Autodesk Inventor part; units mm, degrees
(part 2 of 3)
  line L789 (-22.603724, 22.825849) -> (-22.585944, 20.520291)
  line L790 (-22.585944, 20.520291) -> (-22.128744, 18.275693)
  line L791 (-22.128744, 18.275693) -> (-21.252444, 16.160381)
  line L792 (-21.252444, 16.160381) -> (-19.979904, 14.236585)
  line L793 (-19.979904, 14.236585) -> (-18.328904, 12.570599)
  line L794 (-18.328904, 12.570599) -> (-16.850624, 11.507863)
  line L795 (-16.850624, 11.507863) -> (-16.317224, 11.225415)
  line L796 (7.322556, -11.331563) -> (7.640056, -11.842865)
  line L797 (7.640056, -11.842865) -> (8.788136, -13.249517)
  line L798 (8.788136, -13.249517) -> (10.561056, -14.792059)
  line L799 (10.561056, -14.792059) -> (12.560036, -15.938615)
  line L800 (12.560036, -15.938615) -> (14.726656, -16.675469)
  line L801 (14.726656, -16.675469) -> (16.994876, -16.988397)
  line L802 (16.994876, -16.988397) -> (19.298656, -16.860381)
  line L803 (19.298656, -16.860381) -> (21.569416, -16.274657)
  line L804 (21.569416, -16.274657) -> (23.233116, -15.534501)
  line L805 (23.233116, -15.534501) -> (23.746196, -15.218779)
  line L806 (23.746196, -15.218779) -> (24.254196, -14.903311)
  line L807 (24.254196, -14.903311) -> (25.663896, -13.748373)
  line L808 (25.663896, -13.748373) -> (27.203136, -11.980787)
  line L809 (27.203136, -11.980787) -> (28.351216, -9.979775)
  line L810 (28.351216, -9.979775) -> (29.087816, -7.811885)
  line L811 (29.087816, -7.811885) -> (29.402776, -5.543919)
  line L812 (29.402776, -5.543919) -> (29.275776, -3.240901)
  line L813 (29.275776, -3.240901) -> (28.689036, -0.968617)
  line L814 (28.689036, -0.968617) -> (27.947356, 0.693305)
  line L815 (27.947356, 0.693305) -> (27.629856, 1.204353)
  line L816 (27.629856, 1.204353) -> (27.317436, 1.716925)
  line L817 (27.317436, 1.716925) -> (26.164276, 3.124339)
  line L818 (26.164276, 3.124339) -> (24.396436, 4.666119)
  line L819 (24.396436, 4.666119) -> (22.392376, 5.812675)
  line L820 (22.392376, 5.812675) -> (20.225756, 6.550037)
  line L821 (20.225756, 6.550037) -> (17.957536, 6.862711)
  line L822 (17.957536, 6.862711) -> (15.653756, 6.734441)
  line L823 (15.653756, 6.734441) -> (13.382996, 6.148971)
  line L824 (13.382996, 6.148971) -> (11.721836, 5.407291)
  line L825 (11.721836, 5.407291) -> (11.208756, 5.092077)
  line L826 (11.208756, 5.092077) -> (10.698216, 4.776355)
  line L827 (10.698216, 4.776355) -> (9.291056, 3.622941)
  line L828 (9.291056, 3.622941) -> (7.749276, 1.854847)
  line L829 (7.749276, 1.854847) -> (6.601196, -0.145911)
  line L830 (6.601196, -0.145911) -> (5.864596, -2.313547)
  line L831 (5.864596, -2.313547) -> (5.549636, -4.581767)
  line L832 (5.549636, -4.581767) -> (5.676636, -6.885801)
  line L833 (5.676636, -6.885801) -> (6.263376, -9.157069)
  line L834 (6.263376, -9.157069) -> (7.007596, -10.818991)
  line L835 (7.007596, -10.818991) -> (7.322556, -11.331563)
  line L836 (9.164056, -42.734345) -> (9.174216, -43.335055)
  line L837 (9.174216, -43.335055) -> (9.458696, -45.132105)
  line L838 (9.458696, -45.132105) -> (10.210536, -47.354859)
  line L839 (10.210536, -47.354859) -> (11.358616, -49.355871)
  line L840 (11.358616, -49.355871) -> (12.857216, -51.085103)
  line L841 (12.857216, -51.085103) -> (14.660616, -52.500442)
  line L842 (14.660616, -52.500442) -> (16.712936, -53.550503)
  line L843 (16.712936, -53.550503) -> (18.965916, -54.192641)
  line L844 (18.965916, -54.192641) -> (20.776936, -54.391091)
  line L845 (20.776936, -54.391091) -> (21.378916, -54.377324)
  line L846 (21.378916, -54.377324) -> (21.978356, -54.36216)
  line L847 (21.978356, -54.36216) -> (23.779216, -54.076893)
  line L848 (23.779216, -54.076893) -> (26.001716, -53.327263)
  line L849 (26.001716, -53.327263) -> (27.998156, -52.179361)
  line L850 (27.998156, -52.179361) -> (29.730436, -50.679973)
  line L851 (29.730436, -50.679973) -> (31.145216, -48.878859)
  line L852 (31.145216, -48.878859) -> (32.196776, -46.825777)
  line L853 (32.196776, -46.825777) -> (32.836856, -44.569749)
  line L854 (32.836856, -44.569749) -> (33.034976, -42.760507)
  line L855 (33.034976, -42.760507) -> (33.022276, -42.159543)
  line L856 (33.022276, -42.159543) -> (33.007036, -41.557309)
  line L857 (33.007036, -41.557309) -> (32.722556, -39.760513)
  line L858 (32.722556, -39.760513) -> (31.973256, -37.537759)
  line L859 (31.973256, -37.537759) -> (30.822636, -35.538017)
  line L860 (30.822636, -35.538017) -> (29.324036, -33.807261)
  line L861 (29.324036, -33.807261) -> (27.520636, -32.393497)
  line L862 (27.520636, -32.393497) -> (25.470856, -31.342191)
  line L863 (25.470856, -31.342191) -> (23.215336, -30.699825)
  line L864 (23.215336, -30.699825) -> (21.404316, -30.501451)
  line L865 (21.404316, -30.501451) -> (20.804876, -30.516691)
  line L866 (20.804876, -30.516691) -> (20.202896, -30.530407)
  line L867 (20.202896, -30.530407) -> (18.407116, -30.815395)
  line L868 (18.407116, -30.815395) -> (16.184616, -31.565203)
  line L869 (16.184616, -31.565203) -> (14.183096, -32.713029)
  line L870 (14.183096, -32.713029) -> (12.450816, -34.212391)
  line L871 (12.450816, -34.212391) -> (11.036036, -36.013759)
  line L872 (11.036036, -36.013759) -> (9.984476, -38.066841)
  line L873 (9.984476, -38.066841) -> (9.346936, -40.322869)
  line L874 (9.346936, -40.322869) -> (9.146276, -42.132111)
  line L875 (9.146276, -42.132111) -> (9.164056, -42.734345)
  line L876 (-33.408884, -56.423701) -> (-34.033724, -57.046585)
  line L877 (-34.033724, -57.046585) -> (-36.157164, -58.665759)
  line L878 (-36.157164, -58.665759) -> (-39.200084, -60.267051)
  line L879 (-39.200084, -60.267051) -> (-42.443664, -61.227526)
  line L880 (-42.443664, -61.227526) -> (-45.786304, -61.548633)
  line L881 (-45.786304, -61.548633) -> (-49.128944, -61.227526)
  line L882 (-49.128944, -61.227526) -> (-52.369984, -60.267051)
  line L883 (-52.369984, -60.267051) -> (-55.415444, -58.665759)
  line L884 (-55.415444, -58.665759) -> (-57.536344, -57.046585)
  line L885 (-57.536344, -57.046585) -> (-58.158644, -56.423701)
  line L886 (-58.158644, -56.423701) -> (-58.783484, -55.799445)
  line L887 (-58.783484, -55.799445) -> (-60.404004, -53.677275)
  line L888 (-60.404004, -53.677275) -> (-62.004204, -50.634507)
  line L889 (-62.004204, -50.634507) -> (-62.964324, -47.390673)
  line L890 (-62.964324, -47.390673) -> (-63.286904, -44.048795)
  line L891 (-63.286904, -44.048795) -> (-62.964324, -40.705901)
  line L892 (-62.964324, -40.705901) -> (-62.004204, -37.463337)
  line L893 (-62.004204, -37.463337) -> (-60.404004, -34.419147)
  line L894 (-60.404004, -34.419147) -> (-58.783484, -32.297231)
  line L895 (-58.783484, -32.297231) -> (-58.158644, -31.674169)
  line L896 (-58.158644, -31.674169) -> (-57.536344, -31.049837)
  line L897 (-57.536344, -31.049837) -> (-55.415444, -29.430841)
  line L898 (-55.415444, -29.430841) -> (-52.369984, -27.829625)
  line L899 (-52.369984, -27.829625) -> (-49.128944, -26.868997)
  line L900 (-49.128944, -26.868997) -> (-45.786304, -26.547941)
  line L901 (-45.786304, -26.547941) -> (-42.443664, -26.868997)
  line L902 (-42.443664, -26.868997) -> (-39.200084, -27.829625)
  line L903 (-39.200084, -27.829625) -> (-36.157164, -29.430841)
  line L904 (-36.157164, -29.430841) -> (-34.033724, -31.049837)
  line L905 (-34.033724, -31.049837) -> (-33.408884, -31.674169)
  line L906 (-33.408884, -31.674169) -> (-32.789124, -32.297231)
  line L907 (-32.789124, -32.297231) -> (-31.168604, -34.419147)
  line L908 (-31.168604, -34.419147) -> (-29.568404, -37.463337)
  line L909 (-29.568404, -37.463337) -> (-28.605744, -40.705901)
  line L910 (-28.605744, -40.705901) -> (-28.283164, -44.048795)
  line L911 (-28.283164, -44.048795) -> (-28.605744, -47.390673)
  line L912 (-28.605744, -47.390673) -> (-29.568404, -50.634507)
  line L913 (-29.568404, -50.634507) -> (-31.168604, -53.677275)
  line L914 (-31.168604, -53.677275) -> (-32.789124, -55.799445)
  line L915 (-32.789124, -55.799445) -> (-33.408884, -56.423701)
  line L916 (-54.188624, -52.523861) -> (-53.591724, -51.928561)
  line L917 (-52.384423, -50.722098) -> (-38.507387, -36.843538)
  line L918 (-37.907224, -36.242359) -> (-37.307784, -35.645713)
  line L919 (-37.307784, -52.523861) -> (-37.907224, -51.928561)
  line L920 (-39.111184, -50.721375) -> (-52.989744, -36.844339)
  line L921 (-53.591724, -36.242359) -> (-54.188624, -35.645713)
  line L922 (14.729196, -13.081623) -> (14.482816, -13.060795)
  line L923 (18.978616, -13.034887) -> (18.920196, -13.036157)
  line L924 (18.920196, -13.036157) -> (18.783036, -13.040475)
  line L925 (18.783036, -13.040475) -> (17.419056, -13.063589)
  line L926 (17.419056, -13.063589) -> (17.284436, -13.066637)
  line L927 (17.284436, -13.066637) -> (17.068536, -13.066637)
  line L928 (17.068536, -13.066637) -> (14.942556, -13.099657)
  line L929 (14.942556, -13.099657) -> (14.729196, -13.081623)
  line L930 (-4.793244, -62.273498) -> (-4.752604, -62.254194)
  line L931 (-4.752604, -62.254194) -> (-4.559564, -62.083303)
  line L932 (-4.559564, -62.083303) -> (-4.559564, -62.026814)
  line L933 (-4.559564, -62.026814) -> (-4.559564, -61.924833)
  line L934 (-4.559564, -61.924833) -> (-4.592584, -61.734663)
  line L935 (-52.737996, -50.368564) -> (-38.86096, -36.490004)
  line L936 (-52.03085, -51.075632) -> (-38.153814, -37.197072)
  line L937 (-39.464718, -51.074948) -> (-53.343278, -37.197912)
  line L938 (-38.75765, -50.367802) -> (-52.63621, -36.490766)
  line L939 (-38.153814, -37.197072) -> (-38.86096, -36.490004)
  line L940 (-38.75765, -50.367802) -> (-39.464718, -51.074948)
  line L941 (-52.737996, -50.368564) -> (-52.03085, -51.075632)
  line L942 (-52.63621, -36.490766) -> (-53.343278, -37.197912)
  point P0 (26.657089, 2.522869)
  point P1 (28.23602, 0.046481)
  point P2 (-70.980287, -13.221606)
  point P3 (-70.781416, -10.664974)
  point P4 (-12.499708, 33.522102)
  point P5 (3.750981, -66.644317)
  point P6 (-70.90252, -13.99275)
  point P7 (-14.451188, -45.049937)
  point P8 (-14.090958, -45.024663)
  point P9 (-13.657176, -45.024663)
  point P10 (-12.392664, -45.113647)
  point P11 (-11.715458, -45.204164)
  point P12 (-10.362386, -45.543008)
  point P13 (-9.292197, -45.87547)
  point P14 (-8.154694, -46.428219)
  point P15 (-7.207823, -46.941879)
  point P16 (-6.157427, -47.746057)
  point P17 (-5.380475, -48.386819)
  point P18 (-4.4666, -49.432156)
  point P19 (-3.865434, -50.160677)
  point P20 (-3.113204, -51.481774)
  point P21 (-2.717481, -52.211101)
  point P22 (-2.17304, -53.8869)
  point P23 (-1.982369, -54.500406)
  point P24 (-1.79223, -55.839475)
  point P25 (-1.848254, -58.490356)
  point P26 (-2.230518, -60.213444)
  point P27 (-2.494622, -61.063215)
  point P28 (-4.038829, -63.964888)
  point P29 (-4.410069, -64.414728)
  point P30 (-6.724497, -66.636927)
  point P31 (-6.901029, -66.782518)
  point P32 (-9.069068, -67.970607)
  point P33 (-10.477781, -68.408219)
  point P34 (-16.530305, -68.504563)
  point P35 (-18.074437, -68.024885)
  point P36 (-18.440429, -67.879534)
  point P37 (-19.879408, -67.099838)
  point P38 (-20.383214, -66.812521)
  point P39 (-22.021991, -65.457083)
  point P40 (-22.425656, -64.997007)
  point P41 (-23.403552, -63.814127)
  point P42 (-23.833695, -63.116856)
  point P43 (-24.482688, -61.917917)
  point P44 (-24.794771, -61.149472)
  point P45 (-25.204455, -59.836085)
  point P46 (-25.430368, -58.777249)
  point P47 (-25.521621, -58.095078)
  point P48 (-25.593304, -57.024666)
  point P49 (-25.593304, -56.661836)
  point P50 (-25.56963, -56.17919)
  point P51 (-25.419783, -55.059031)
  point P52 (-25.301336, -54.389917)
  point P53 (-24.905044, -53.119435)
  point P54 (-24.588154, -52.192295)
  point P55 (-24.111863, -51.312447)
  point P56 (-21.065728, -47.667296)
  point P57 (-20.493311, -47.193856)
  point P58 (-19.456689, -46.586467)
  point P59 (-18.526645, -46.082568)
  point P60 (-17.578172, -45.736339)
  point P61 (-16.261766, -45.327388)
  point P62 (-15.697902, -45.216811)
  point P63 (-32.132489, 34.644603)
  point P64 (-35.142865, 34.293968)
  point P65 (-69.1257, 0.22919)
  point P66 (-70.299173, -6.530143)
  point P67 (-70.363625, -7.082766)
  point P68 (15.877196, -62.416221)
  point P69 (17.047598, -61.83976)
  point P70 (34.387532, -28.646734)
  point P71 (34.353637, -28.003816)
  point P72 (9.452137, 19.037752)
  point P73 (8.27439, 20.009449)
  point P74 (-36.407377, 19.257413)
  point P75 (-37.127948, 15.741932)
  point P76 (-37.16308, 15.662676)
  point P77 (-38.109165, 13.74007)
  point P78 (-38.289337, 13.473296)
  point P79 (-39.40199, 12.011768)
  point P80 (-39.793143, 11.604587)
  point P81 (-40.934583, 10.582054)
  point P82 (-41.579317, 10.105711)
  point P83 (-42.720858, 9.425909)
  point P84 (-43.526766, 9.019144)
  point P85 (-44.809198, 8.564772)
  point P86 (-45.680707, 8.299855)
  point P87 (-46.652701, 8.12955)
  point P88 (-47.350022, 8.023598)
  point P89 (-47.938503, 7.999615)
  point P90 (-48.575756, 7.994027)
  point P91 (-49.709686, 8.101058)
  point P92 (-50.388844, 8.190593)
  point P93 (-51.657409, 8.529209)
  point P94 (-52.659665, 8.831052)
  point P95 (-53.784254, 9.384239)
  point P96 (-54.690294, 9.860171)
  point P97 (-55.678233, 10.610482)
  point P98 (-56.476925, 11.244335)
  point P99 (-57.323583, 12.191296)
  point P100 (-57.971801, 12.941087)
  point P101 (-58.65977, 14.095394)
  point P102 (-59.126949, 14.900308)
  point P103 (-59.690576, 16.492921)
  point P104 (-59.895339, 17.084166)
  point P105 (-60.235804, 19.618519)
  point P106 (-60.199445, 20.635684)
  point P107 (-60.139424, 21.274863)
  point P108 (-44.404458, 31.181517)
  point P109 (-43.908, 31.00537)
  point P110 (-42.823468, 30.47202)
  point P111 (-41.847578, 29.942526)
  point P112 (-40.939105, 29.251808)
  point P113 (-40.093943, 28.56811)
  point P114 (-39.285921, 27.663664)
  point P115 (-38.623993, 26.888971)
  point P116 (-37.922645, 25.712215)
  point P117 (-37.482851, 24.950917)
  point P118 (-36.898866, 23.305176)
  point P119 (-36.384985, 20.504957)
  point P120 (-36.383619, 20.472644)
  point P121 (0.598463, 25.558408)
  point P122 (1.111089, 23.222486)
  point P123 (1.165157, 21.742405)
  point P124 (1.172107, 20.840768)
  point P125 (0.899345, 19.25247)
  point P126 (0.747134, 18.449733)
  point P127 (0.310087, 17.242941)
  point P128 (0.104117, 16.687319)
  point P129 (-0.468312, 15.612618)
  point P130 (-0.902103, 15.008527)
  point P131 (-1.849187, 13.821679)
  point P132 (-2.505593, 13.172266)
  point P133 (-4.28973, 11.767595)
  point P134 (-4.848146, 11.398244)
  point P135 (-7.446953, 10.303356)
  point P136 (-8.75938, 10.036862)
  point P137 (-9.575058, 9.890829)
  point P138 (-12.609908, 10.030609)
  point P139 (-14.415298, 10.433739)
  point P140 (-14.788027, 10.572332)
  point P141 (-17.365174, 11.877773)
  point P142 (-19.365663, 13.616768)
  point P143 (-22.450919, 23.631804)
  point P144 (-21.72057, 26.328829)
  point P145 (-19.675191, 29.606141)
  point P146 (-18.975433, 30.299284)
  point P147 (-17.882197, 31.264757)
  point P148 (-16.576816, 32.129378)
  point P149 (-16.244236, 32.331452)
  point P150 (-15.367761, 32.6933)
  point P151 (29.198236, -7.016772)
  point P152 (28.443584, -9.707927)
  point P153 (27.76169, -11.007272)
  point P154 (27.305264, -11.802786)
  point P155 (26.260434, -13.063339)
  point P156 (25.715234, -13.689419)
  point P157 (24.776107, -14.47572)
  point P158 (21.082473, -16.40026)
  point P159 (19.905491, -16.703853)
  point P160 (18.941227, -16.880243)
  point P161 (15.34623, -16.760947)
  point P162 (14.597597, -16.631577)
  point P163 (14.035431, -16.440388)
  point P164 (11.968166, -15.599136)
  point P165 (11.229638, -15.175538)
  point P166 (9.490883, -13.860947)
  point P167 (8.941532, -13.382981)
  point P168 (7.614367, -11.801495)
  point P169 (7.165811, -11.076474)
  point P170 (6.963602, -10.720747)
  point P171 (6.517957, -9.725576)
  point P172 (6.225389, -9.010022)
  point P173 (5.995587, -8.120458)
  point P174 (5.664674, -6.668788)
  point P175 (5.656568, -6.521727)
  point P176 (8.809351, 3.070527)
  point P177 (9.246444, 3.57178)
  point P178 (9.815194, 4.052564)
  point P179 (10.647556, 4.73483)
  point P180 (11.165512, 5.065335)
  point P181 (11.589468, 5.325969)
  point P182 (13.830183, 6.264269)
  point P183 (14.964707, 6.556783)
  point P184 (16.016046, 6.754612)
  point P185 (19.962259, 6.58636)
  point P186 (20.621162, 6.415469)
  point P187 (28.298949, -51.919007)
  point P188 (27.202918, -52.636602)
  point P189 (25.423153, -53.522407)
  point P190 (24.575291, -53.808384)
  point P191 (22.13415, -54.337482)
  point P192 (21.979406, -54.361994)
  point P193 (20.689085, -54.381464)
  point P194 (19.560515, -54.257796)
  point P195 (18.877281, -54.167378)
  point P196 (17.574428, -53.796043)
  point P197 (16.628337, -53.507219)
  point P198 (15.440099, -52.899261)
  point P199 (14.594831, -52.448813)
  dimension "d36" = 0.5
  dimension "d37" = 0.5
  dimension "d38" = 0.5
  dimension "d39" = 0.5
  constraints: 1886 end point, 4 parallel, 4 perpendicular
  measures "d36" distance between parallel lines of L917 L935
  measures "d37" distance between parallel lines of L917 L936
  measures "d38" distance between parallel lines of L920 L937
  measures "d39" distance between parallel lines of L920 L938
sketch "Sketch1 outline for Extrusion3" plane through (0, 0, 0) normal (1, 0, 0) x (0, 1, 0)
  line L0 (-8.194304, 39.472755) -> (-13.782304, 40.987103)
  line L1 (-13.782304, 40.987103) -> (-19.456664, 41.986085)
  line L2 (-19.456664, 41.986085) -> (-25.166584, 42.447603)
  line L3 (-25.166584, 42.447603) -> (-30.851104, 42.347019)
  line L4 (-30.851104, 42.347019) -> (-36.469584, 41.662235)
  line L5 (-36.469584, 41.662235) -> (-41.958524, 40.369883)
  line L6 (-41.958524, 40.369883) -> (-47.272204, 38.443293)
  line L7 (-47.272204, 38.443293) -> (-52.354744, 35.861891)
  line L8 (-52.354744, 35.861891) -> (-57.155344, 32.600277)
  line L9 (-57.155344, 32.600277) -> (-60.571644, 29.694009)
  line L10 (-60.571644, 29.694009) -> (-61.618124, 28.635591)
  line L11 (-61.618124, 28.635591) -> (-62.369964, 27.748115)
  line L12 (-62.369964, 27.748115) -> (-64.437524, 24.924905)
  line L13 (-64.437524, 24.924905) -> (-66.926724, 20.862175)
  line L14 (-66.926724, 20.862175) -> (-69.085724, 16.492359)
  line L15 (-69.085724, 16.492359) -> (-70.922144, 11.855589)
  line L16 (-70.922144, 11.855589) -> (-72.438524, 6.993521)
  line L17 (-72.438524, 6.993521) -> (-73.637404, 1.946033)
  line L18 (-73.637404, 1.946033) -> (-74.521324, -3.242425)
  line L19 (-74.521324, -3.242425) -> (-75.095364, -8.532737)
  line L20 (-75.095364, -8.532737) -> (-75.362064, -13.882231)
  line L21 (-75.362064, -13.882231) -> (-75.329044, -19.251029)
  line L22 (-75.329044, -19.251029) -> (-74.993764, -24.596459)
  line L23 (-74.993764, -24.596459) -> (-74.363844, -29.878389)
  line L24 (-74.363844, -29.878389) -> (-73.441824, -35.053131)
  line L25 (-73.441824, -35.053131) -> (-72.230244, -40.081569)
  line L26 (-72.230244, -40.081569) -> (-70.731644, -44.921285)
  line L27 (-70.731644, -44.921285) -> (-69.441324, -48.395243)
  line L28 (-69.441324, -48.395243) -> (-68.953644, -49.530877)
  line L29 (-68.953644, -49.530877) -> (-68.570104, -50.426481)
  line L30 (-68.570104, -50.426481) -> (-67.221364, -53.028203)
  line L31 (-67.221364, -53.028203) -> (-65.128404, -56.283137)
  line L32 (-65.128404, -56.283137) -> (-62.702704, -59.270736)
  line L33 (-62.702704, -59.270736) -> (-59.969664, -61.964812)
  line L34 (-59.969664, -61.964812) -> (-56.959764, -64.341922)
  line L35 (-56.959764, -64.341922) -> (-53.695864, -66.375903)
  line L36 (-53.695864, -66.375903) -> (-50.208444, -68.044709)
  line L37 (-50.208444, -68.044709) -> (-47.455084, -69.056162)
  line L38 (-47.455084, -69.056162) -> (-46.517824, -69.322125)
  line L39 (-46.517824, -69.322125) -> (-45.420544, -69.633606)
  line L40 (-45.420544, -69.633606) -> (-42.082984, -70.421793)
  line L41 (-42.082984, -70.421793) -> (-37.378904, -71.292734)
  line L42 (-37.378904, -71.292734) -> (-32.453844, -71.932153)
  line L43 (-32.453844, -71.932153) -> (-27.361144, -72.340026)
  line L44 (-27.361144, -72.340026) -> (-22.146524, -72.515058)
  line L45 (-22.146524, -72.515058) -> (-16.860784, -72.457197)
  line L46 (-16.860784, -72.457197) -> (-11.554724, -72.16502)
  line L47 (-11.554724, -72.16502) -> (-6.284224, -71.638631)
  line L48 (-6.284224, -71.638631) -> (-1.092464, -70.875183)
  line L49 (-1.092464, -70.875183) -> (3.969756, -69.877496)
  line L50 (3.969756, -69.877496) -> (8.849096, -68.641405)
  line L51 (8.849096, -68.641405) -> (13.494756, -67.168282)
  line L52 (13.494756, -67.168282) -> (17.863556, -65.455356)
  line L53 (17.863556, -65.455356) -> (21.894536, -63.504078)
  line L54 (21.894536, -63.504078) -> (25.547056, -61.312972)
  line L55 (25.547056, -61.312972) -> (28.000696, -59.535328)
  line L56 (28.000696, -59.535328) -> (28.767776, -58.882116)
  line L57 (28.767776, -58.882116) -> (29.755836, -57.854102)
  line L58 (29.755836, -57.854102) -> (32.450776, -54.506864)
  line L59 (32.450776, -54.506864) -> (35.420036, -49.840757)
  line L60 (35.420036, -49.840757) -> (37.706036, -44.926619)
  line L61 (37.706036, -44.926619) -> (39.346876, -39.811313)
  line L62 (39.346876, -39.811313) -> (40.370496, -34.537511)
  line L63 (40.370496, -34.537511) -> (40.814996, -29.152457)
  line L64 (40.814996, -29.152457) -> (40.713396, -23.700601)
  line L65 (40.713396, -23.700601) -> (40.091096, -18.228679)
  line L66 (40.091096, -18.228679) -> (38.991276, -12.778347)
  line L67 (38.991276, -12.778347) -> (37.441876, -7.398373)
  line L68 (37.441876, -7.398373) -> (35.475916, -2.131937)
  line L69 (35.475916, -2.131937) -> (33.131496, 2.976765)
  line L70 (33.131496, 2.976765) -> (30.439096, 7.879727)
  line L71 (30.439096, 7.879727) -> (27.429196, 12.533515)
  line L72 (27.429196, 12.533515) -> (24.139896, 16.892155)
  line L73 (24.139896, 16.892155) -> (21.521156, 19.942949)
  line L74 (21.521156, 19.942949) -> (20.599136, 20.910435)
  line L75 (20.599136, 20.910435) -> (19.661876, 21.984093)
  line L76 (19.661876, 21.984093) -> (16.629116, 25.015583)
  line L77 (16.629116, 25.015583) -> (12.257776, 28.747097)
  line L78 (12.257776, 28.747097) -> (7.535916, 32.082371)
  line L79 (7.535916, 32.082371) -> (2.519416, 34.996513)
  line L80 (2.519416, 34.996513) -> (-2.738384, 37.468949)
  line L81 (-2.738384, 37.468949) -> (-8.194304, 39.472755)
extrude "Extrusion3" add sketch "Sketch1 outline for Extrusion3" along normal blind 0.25
sketch "Sketch1 outline for Extrusion17" plane through (0, 0, 0) normal (1, 0, 0) x (0, 1, 0)
  line L0 (6.979656, 20.566011) -> (4.947656, 20.520291)
  line L1 (8.27439, 20.009449) -> (6.979656, 20.566011)
  line L2 (9.452137, 19.037752) -> (8.27439, 20.009449)
  line L3 (13.913856, 14.827643) -> (9.452137, 19.037752)
  line L4 (14.343116, 14.406003) -> (13.913856, 14.827643)
  line L5 (14.726656, 14.025765) -> (14.343116, 14.406003)
  line L6 (15.473416, 12.470015) -> (14.726656, 14.025765)
  line L7 (15.496276, 10.350639) -> (15.473416, 12.470015)
  line L8 (14.510756, 8.472309) -> (15.496276, 10.350639)
  line L9 (13.139156, 7.424813) -> (14.510756, 8.472309)
  line L10 (12.620996, 7.259459) -> (13.139156, 7.424813)
  line L11 (12.430496, 7.198753) -> (12.620996, 7.259459)
  line L12 (10.624556, 6.409321) -> (12.430496, 7.198753)
  line L13 (10.456916, 6.310261) -> (10.624556, 6.409321)
  line L14 (9.839696, 5.942215) -> (10.456916, 6.310261)
  line L15 (8.153136, 4.555883) -> (9.839696, 5.942215)
  line L16 (6.326876, 2.359291) -> (8.153136, 4.555883)
  line L17 (5.018776, -0.196711) -> (6.326876, 2.359291)
  line L18 (4.376156, -2.312531) -> (5.018776, -0.196711)
  line L19 (4.266936, -3.032875) -> (4.376156, -2.312531)
  line L20 (4.160256, -3.691751) -> (4.266936, -3.032875)
  line L21 (4.241536, -6.999085) -> (4.160256, -3.691751)
  line L22 (5.110216, -10.191611) -> (4.241536, -6.999085)
  line L23 (5.399776, -10.793845) -> (5.110216, -10.191611)
  line L24 (5.811256, -11.649825) -> (5.399776, -10.793845)
  line L25 (7.523216, -13.988403) -> (5.811256, -11.649825)
  line L26 (10.362936, -16.391751) -> (7.523216, -13.988403)
  line L27 (13.741136, -17.904829) -> (10.362936, -16.391751)
  line L28 (16.550376, -18.431117) -> (13.741136, -17.904829)
  line L29 (17.487636, -18.431117) -> (16.550376, -18.431117)
  line L30 (18.399496, -18.431117) -> (17.487636, -18.431117)
  line L31 (21.124916, -17.922863) -> (18.399496, -18.431117)
  line L32 (23.969716, -16.763607) -> (21.124916, -17.922863)
  line L33 (24.498036, -16.438487) -> (23.969716, -16.763607)
  line L34 (24.622496, -16.361525) -> (24.498036, -16.438487)
  line L35 (25.793436, -15.530437) -> (24.622496, -16.361525)
  line L36 (25.905196, -15.440775) -> (25.793436, -15.530437)
  line L37 (26.321756, -15.103209) -> (25.905196, -15.440775)
  line L38 (27.919416, -14.524597) -> (26.321756, -15.103209)
  line L39 (30.009836, -14.684363) -> (27.919416, -14.524597)
  line L40 (31.772596, -15.796375) -> (30.009836, -14.684363)
  line L41 (32.697156, -17.218267) -> (31.772596, -15.796375)
  line L42 (32.821616, -17.736681) -> (32.697156, -17.218267)
  line L43 (33.045136, -18.676481) -> (32.821616, -17.736681)
  line L44 (33.901116, -23.420947) -> (33.045136, -18.676481)
  line L45 (34.353637, -28.003816) -> (33.901116, -23.420947)
  line L46 (34.387532, -28.646734) -> (34.353637, -28.003816)
  line L47 (34.404036, -29.167697) -> (34.387532, -28.646734)
  line L48 (34.404036, -29.179889) -> (34.404036, -29.167697)
  line L49 (34.409116, -29.328987) -> (34.404036, -29.179889)
  line L50 (34.409116, -29.378263) -> (34.409116, -29.328987)
  line L51 (34.409116, -29.608641) -> (34.409116, -29.378263)
  line L52 (34.274496, -30.304347) -> (34.409116, -29.608641)
  line L53 (33.906196, -31.098097) -> (34.274496, -30.304347)
  line L54 (33.347396, -31.737669) -> (33.906196, -31.098097)
  line L55 (32.641276, -32.201981) -> (33.347396, -31.737669)
  line L56 (31.838636, -32.469189) -> (32.641276, -32.201981)
  line L57 (30.982656, -32.517703) -> (31.838636, -32.469189)
  line L58 (30.121596, -32.324663) -> (30.982656, -32.517703)
  line L59 (29.484056, -32.011735) -> (30.121596, -32.324663)
  line L60 (29.298636, -31.872289) -> (29.484056, -32.011735)
  line L61 (29.090356, -31.716841) -> (29.298636, -31.872289)
  line L62 (27.937196, -30.970081) -> (29.090356, -31.716841)
  line L63 (26.618936, -30.272597) -> (27.937196, -30.970081)
  line L64 (26.329376, -30.143057) -> (26.618936, -30.272597)
  line L65 (25.922976, -29.961447) -> (26.329376, -30.143057)
  line L66 (23.789376, -29.338385) -> (25.922976, -29.961447)
  line L67 (21.767536, -29.080575) -> (23.789376, -29.338385)
  line L68 (21.096976, -29.080575) -> (21.767536, -29.080575)
  line L69 (21.013156, -29.080575) -> (21.096976, -29.080575)
  line L70 (20.797256, -29.083369) -> (21.013156, -29.080575)
  line L71 (20.769316, -29.084639) -> (20.797256, -29.083369)
  line L72 (20.058116, -29.101403) -> (20.769316, -29.084639)
  line L73 (17.929596, -29.458273) -> (20.058116, -29.101403)
  line L74 (15.313396, -30.394009) -> (17.929596, -29.458273)
  line L75 (12.984216, -31.825807) -> (15.313396, -30.394009)
  line L76 (11.000476, -33.687373) -> (12.984216, -31.825807)
  line L77 (9.435836, -35.914445) -> (11.000476, -33.687373)
  line L78 (8.338556, -38.437681) -> (9.435836, -35.914445)
  line L79 (7.784836, -41.193581) -> (8.338556, -38.437681)
  line L80 (7.739116, -43.394491) -> (7.784836, -41.193581)
  line L81 (7.830556, -44.115089) -> (7.739116, -43.394491)
  line L82 (7.894056, -44.646965) -> (7.830556, -44.115089)
  line L83 (8.338556, -46.212367) -> (7.894056, -44.646965)
  line L84 (9.291056, -48.428263) -> (8.338556, -46.212367)
  line L85 (10.533116, -50.500903) -> (9.291056, -48.428263)
  line L86 (11.526256, -51.794881) -> (10.533116, -50.500903)
  line L87 (11.912336, -52.17522) -> (11.526256, -51.794881)
  line L88 (12.143476, -52.408088) -> (11.912336, -52.17522)
  line L89 (13.385536, -53.463661) -> (12.143476, -52.408088)
  line L90 (14.762216, -54.2726) -> (13.385536, -53.463661)
  line L91 (15.061936, -54.381464) -> (14.762216, -54.2726)
  line L92 (15.107656, -54.398) -> (15.061936, -54.381464)
  line L93 (15.580096, -54.561982) -> (15.107656, -54.398)
  line L94 (15.625816, -54.578518) -> (15.580096, -54.561982)
  line L95 (16.202396, -54.768662) -> (15.625816, -54.578518)
  line L96 (17.693376, -56.064037) -> (16.202396, -54.768662)
  line L97 (18.516336, -58.308863) -> (17.693376, -56.064037)
  line L98 (18.046436, -60.654274) -> (18.516336, -58.308863)
  line L99 (17.047598, -61.83976) -> (18.046436, -60.654274)
  line L100 (15.877196, -62.416221) -> (17.047598, -61.83976)
  line L101 (13.459196, -63.606033) -> (15.877196, -62.416221)
  line L102 (7.789916, -65.571104) -> (13.459196, -63.606033)
  line L103 (3.750981, -66.644317) -> (7.789916, -65.571104)
  line L104 (2.918196, -66.687333) -> (3.750981, -66.644317)
  line L105 (1.803136, -66.483396) -> (2.918196, -66.687333)
  line L106 (0.812536, -66.003819) -> (1.803136, -66.483396)
  line L107 (-0.015504, -65.294143) -> (0.812536, -66.003819)
  line L108 (-0.647964, -64.39704) -> (-0.015504, -65.294143)
  line L109 (-1.031504, -63.358002) -> (-0.647964, -64.39704)
  line L110 (-1.140724, -62.22247) -> (-1.031504, -63.358002)
  line L111 (-1.021344, -61.318484) -> (-1.140724, -62.22247)
  line L112 (-0.929904, -61.034639) -> (-1.021344, -61.318484)
  line L113 (-0.820684, -60.695625) -> (-0.929904, -61.034639)
  line L114 (-0.439684, -58.935862) -> (-0.820684, -60.695625)
  line L115 (-0.287284, -57.101703) -> (-0.439684, -58.935862)
  line L116 (-0.294904, -56.726875) -> (-0.287284, -57.101703)
  line L117 (-0.305064, -55.986871) -> (-0.294904, -56.726875)
  line L118 (-0.678444, -53.775116) -> (-0.305064, -55.986871)
  line L119 (-1.676664, -51.086627) -> (-0.678444, -53.775116)
  line L120 (-3.208284, -48.720363) -> (-1.676664, -51.086627)
  line L121 (-5.194564, -46.734591) -> (-3.208284, -48.720363)
  line L122 (-7.549144, -45.190017) -> (-5.194564, -46.734591)
  line L123 (-10.198364, -44.146839) -> (-7.549144, -45.190017)
  line L124 (-13.055864, -43.661699) -> (-10.198364, -44.146839)
  line L125 (-15.308844, -43.683797) -> (-13.055864, -43.661699)
  line L126 (-16.042904, -43.796827) -> (-15.308844, -43.683797)
  line L127 (-16.268964, -43.831117) -> (-16.042904, -43.796827)
  line L128 (-18.295884, -44.302541) -> (-16.268964, -43.831117)
  line L129 (-18.481304, -44.361723) -> (-18.295884, -44.302541)
  line L130 (-18.712444, -44.434875) -> (-18.481304, -44.361723)
  line L131 (-19.438884, -44.556033) -> (-18.712444, -44.434875)
  line L132 (-20.378684, -44.539523) -> (-19.438884, -44.556033)
  line L133 (-21.275304, -44.324639) -> (-20.378684, -44.539523)
  line L134 (-22.095724, -43.931701) -> (-21.275304, -44.324639)
  line L135 (-22.817084, -43.375187) -> (-22.095724, -43.931701)
  line L136 (-23.406364, -42.672369) -> (-22.817084, -43.375187)
  line L137 (-23.835624, -41.840011) -> (-23.406364, -42.672369)
  line L138 (-24.051524, -41.134145) -> (-23.835624, -41.840011)
  line L139 (-24.082004, -40.894623) -> (-24.051524, -41.134145)
  line L140 (-24.209004, -40.036103) -> (-24.082004, -40.894623)
  line L141 (-24.854164, -37.500675) -> (-24.209004, -40.036103)
  line L142 (-26.147024, -34.259381) -> (-24.854164, -37.500675)
  line L143 (-27.955504, -31.241353) -> (-26.147024, -34.259381)
  line L144 (-29.631904, -29.148139) -> (-27.955504, -31.241353)
  line L145 (-30.259284, -28.521013) -> (-29.631904, -29.148139)
  line L146 (-31.021284, -27.757489) -> (-30.259284, -28.521013)
  line L147 (-33.607004, -25.767907) -> (-31.021284, -27.757489)
  line L148 (-37.376364, -23.753179) -> (-33.607004, -25.767907)
  line L149 (-41.463224, -22.514167) -> (-37.376364, -23.753179)
  line L150 (-44.699184, -22.094051) -> (-41.463224, -22.514167)
  line L151 (-45.778684, -22.094051) -> (-44.699184, -22.094051)
  line L152 (-46.916604, -22.094051) -> (-45.778684, -22.094051)
  line L153 (-50.335444, -22.565475) -> (-46.916604, -22.094051)
  line L154 (-53.980344, -23.662247) -> (-50.335444, -22.565475)
  line L155 (-54.686464, -23.975175) -> (-53.980344, -23.662247)
  line L156 (-55.402744, -24.282261) -> (-54.686464, -23.975175)
  line L157 (-57.719224, -24.823789) -> (-55.402744, -24.282261)
  line L158 (-60.711344, -24.846141) -> (-57.719224, -24.823789)
  line L159 (-63.533284, -24.125289) -> (-60.711344, -24.846141)
  line L160 (-66.070744, -22.747085) -> (-63.533284, -24.125289)
  line L161 (-68.199264, -20.800175) -> (-66.070744, -22.747085)
  line L162 (-69.799464, -18.366347) -> (-68.199264, -20.800175)
  line L163 (-70.746884, -15.536025) -> (-69.799464, -18.366347)
  line L164 (-70.90252, -13.99275) -> (-70.746884, -15.536025)
  line L165 (-70.363625, -7.082766) -> (-70.90252, -13.99275)
  line L166 (-70.299173, -6.530143) -> (-70.363625, -7.082766)
  line L167 (-69.1257, 0.22919) -> (-70.299173, -6.530143)
  line L168 (-67.795404, 5.604649) -> (-69.1257, 0.22919)
  line L169 (-66.380624, 9.963035) -> (-67.795404, 5.604649)
  line L170 (-65.816744, 11.379847) -> (-66.380624, 9.963035)
  line L171 (-65.814204, 11.387975) -> (-65.816744, 11.379847)
  line L172 (-65.788804, 11.460111) -> (-65.814204, 11.387975)
  line L173 (-65.786264, 11.466715) -> (-65.788804, 11.460111)
  line L174 (-65.623704, 11.930011) -> (-65.786264, 11.466715)
  line L175 (-64.597544, 13.127113) -> (-65.623704, 11.930011)
  line L176 (-62.817004, 13.871333) -> (-64.597544, 13.127113)
  line L177 (-60.906924, 13.634605) -> (-62.817004, 13.871333)
  line L178 (-59.606444, 12.751193) -> (-60.906924, 13.634605)
  line L179 (-59.329584, 12.347333) -> (-59.606444, 12.751193)
  line L180 (-58.885084, 11.698109) -> (-59.329584, 12.347333)
  line L181 (-57.236624, 9.963035) -> (-58.885084, 11.698109)
  line L182 (-54.635664, 8.138553) -> (-57.236624, 9.963035)
  line L183 (-51.625764, 6.972947) -> (-54.635664, 8.138553)
  line L184 (-49.141644, 6.560959) -> (-51.625764, 6.972947)
  line L185 (-48.313604, 6.560959) -> (-49.141644, 6.560959)
  line L186 (-48.222164, 6.560959) -> (-48.313604, 6.560959)
  line L187 (-47.975784, 6.566293) -> (-48.222164, 6.560959)
  line L188 (-47.945304, 6.566293) -> (-47.975784, 6.566293)
  line L189 (-47.196004, 6.587121) -> (-47.945304, 6.566293)
  line L190 (-43.571424, 7.422019) -> (-47.196004, 6.587121)
  line L191 (-40.302444, 9.184525) -> (-43.571424, 7.422019)
  line L192 (-39.730944, 9.669665) -> (-40.302444, 9.184525)
  line L193 (-39.141664, 10.168521) -> (-39.730944, 9.669665)
  line L194 (-37.597344, 11.928487) -> (-39.141664, 10.168521)
  line L195 (-36.065724, 14.539861) -> (-37.597344, 11.928487)
  line L196 (-35.174184, 17.415649) -> (-36.065724, 14.539861)
  line L197 (-34.920184, 19.703427) -> (-35.174184, 17.415649)
  line L198 (-34.948124, 20.461109) -> (-34.920184, 19.703427)
  line L199 (-34.976064, 21.142083) -> (-34.948124, 20.461109)
  line L200 (-35.682184, 24.350103) -> (-34.976064, 21.142083)
  line L201 (-37.071564, 27.224621) -> (-35.682184, 24.350103)
  line L202 (-37.442404, 27.737193) -> (-37.071564, 27.224621)
  line L203 (-37.759904, 28.180931) -> (-37.442404, 27.737193)
  line L204 (-38.222184, 29.862411) -> (-37.759904, 28.180931)
  line L205 (-37.836104, 31.969087) -> (-38.222184, 29.862411)
  line L206 (-36.482284, 33.643455) -> (-37.836104, 31.969087)
  line L207 (-35.142865, 34.293968) -> (-36.482284, 33.643455)
  line L208 (-32.132489, 34.644603) -> (-35.142865, 34.293968)
  line L209 (-26.421344, 34.584525) -> (-32.132489, 34.644603)
  line L210 (-25.847304, 34.540583) -> (-26.421344, 34.584525)
  line L211 (-25.324064, 34.500705) -> (-25.847304, 34.540583)
  line L212 (-23.789904, 33.829637) -> (-25.324064, 34.500705)
  line L213 (-22.418304, 32.292937) -> (-23.789904, 33.829637)
  line L214 (-21.905224, 30.288115) -> (-22.418304, 32.292937)
  line L215 (-22.192244, 28.632797) -> (-21.905224, 30.288115)
  line L216 (-22.446244, 28.167215) -> (-22.192244, 28.632797)
  line L217 (-22.453864, 28.157563) -> (-22.446244, 28.167215)
  line L218 (-22.509744, 28.050121) -> (-22.453864, 28.157563)
  line L219 (-22.512284, 28.039199) -> (-22.509744, 28.050121)
  line L220 (-22.931384, 27.252053) -> (-22.512284, 28.039199)
  line L221 (-24.026124, 23.047591) -> (-22.931384, 27.252053)
  line L222 (-23.756884, 18.711049) -> (-24.026124, 23.047591)
  line L223 (-23.497804, 17.856593) -> (-23.756884, 18.711049)
  line L224 (-23.307304, 17.229721) -> (-23.497804, 17.856593)
  line L225 (-22.484344, 15.418955) -> (-23.307304, 17.229721)
  line L226 (-21.039084, 13.258177) -> (-22.484344, 15.418955)
  line L227 (-19.192504, 11.424043) -> (-21.039084, 13.258177)
  line L228 (-17.574524, 10.270375) -> (-19.192504, 11.424043)
  line L229 (-16.992864, 9.961765) -> (-17.574524, 10.270375)
  line L230 (-16.512804, 9.705733) -> (-16.992864, 9.961765)
  line L231 (-13.949944, 8.793365) -> (-16.512804, 9.705733)
  line L232 (-11.531864, 8.392299) -> (-13.949944, 8.793365)
  line L233 (-10.726684, 8.392299) -> (-11.531864, 8.392299)
  line L234 (-9.822444, 8.392299) -> (-10.726684, 8.392299)
  line L235 (-7.117344, 8.885821) -> (-9.822444, 8.392299)
  line L236 (-3.833124, 10.298315) -> (-7.117344, 8.885821)
  line L237 (-1.041664, 12.530721) -> (-3.833124, 10.298315)
  line L238 (0.660136, 14.687181) -> (-1.041664, 12.530721)
  line L239 (1.084316, 15.482455) -> (0.660136, 14.687181)
  line L240 (1.183376, 15.664319) -> (1.084316, 15.482455)
  line L241 (1.965696, 17.528933) -> (1.183376, 15.664319)
  line L242 (2.026656, 17.717655) -> (1.965696, 17.528933)
  line L243 (2.181596, 18.213463) -> (2.026656, 17.717655)
  line L244 (3.169656, 19.536549) -> (2.181596, 18.213463)
  line L245 (4.947656, 20.520291) -> (3.169656, 19.536549)
extrude "Extrusion17" add sketch "Sketch1 outline for Extrusion17" along normal blind 0.5